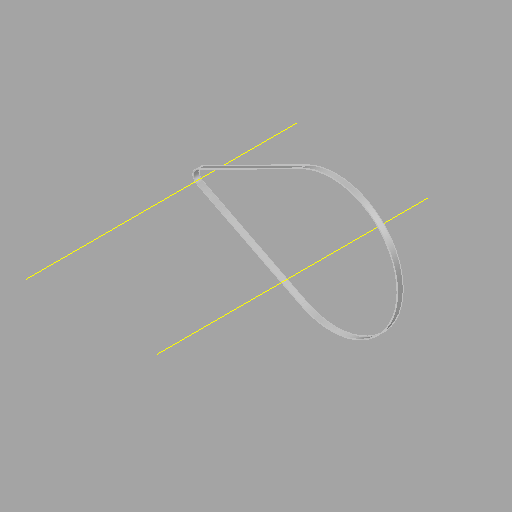
# Autodesk Inventor part: Synchronous Belt
Saved by Autodesk Inventor 2025.2 (Build 292293000, 293)
## iProperties
CustomPartVersion: 1
Created: 2025-04-10
Part Number: Synchronous Belt
Material: Rubber
Document SubType Name: Modeling
Designer: Tiago
Density: 1 g/cm^3
Appearance: Rubber - Black - Version 1.1
Author: Tiago
Autodesk Inventor part; units mm, degrees
ref_plane "YZ Plane" through (0, 0, 0) normal (1, 0, 0) x (0, 1, 0)
ref_plane "XZ Plane" through (0, 0, 0) normal (0, 1, 0) x (-1, 0, 0)
ref_plane "XY Plane" through (0, 0, 0) normal (0, 0, 1) x (1, 0, 0)
sketch "Sketch Path" plane through (0, 0, 0) normal (0, 0, 1) x (1, 0, 0)
  arc A0 (-3.5983, 7.0977) -> (-3.5983, -7.0977) centre (0, 0) ccw
  arc A1 (108.4052, -63.8797) -> (108.4052, 63.8797) centre (140.79, 0) ccw
  line L0 (108.4052, -63.8797) -> (-3.5983, -7.0977)
  line L1 (-3.5983, 7.0977) -> (108.4052, 63.8797)
  constraints: 4 end point, 4 point on circle, 2 centre point
ref_plane "Cross Section Plane" through (-3.5983, -7.0977, 0) normal (0.8919283, -0.4521768, 0) x (0, 0, 1)
ref_plane "Work Plane2" through (0, 0, 0) normal (-1, 0, 0) x (0, 0, 1)
ref_plane "Work Plane3" through (140.79, 0, 0) normal (-0.8960525, -0.443948, 0) x (0, 0, 1)
sketch "Cross Section" plane through (-3.5983, -7.0977, 0) normal (0.8919283, -0.4521768, 0) x (0, 0, 1)
  line L0 (-3, 0.3) -> (3, 0.3)
  line L1 (3, 0.3) -> (3, -0.3)
  line L2 (3, -0.3) -> (-3, -0.3)
  line L3 (-3, -0.3) -> (-3, 0.3)
  line L4 (-3, 0) -> (3, 0) construction
  point P0 (0, 0)
  point P1 (0, 0)
  dimension "d0" = 6
  dimension "d4" = 0.3
  dimension "d5" = 0.3
  constraints: 10 end point, 3 midpoint, 2 parallel, 1 coincident, 1 horizontal, 1 perpendicular, 1 other
  measures "d0" distance between parallel lines of L1 L3
  measures "d4" distance between parallel lines of L2 L4
  measures "d5" distance between parallel lines of L4 L0
sweep "Belt" add profiles "Cross Section" path "Sketch Path" path curves L1 A1 L0 A0
equation "\"d0\" = da_B"
equation "\"d4\" = da_a"
equation "\"d5\" = da_a2"
equation "\"da_B\" = 6"
equation "\"da_pb\" = 2.5"
equation "\"da_L\" = 560.89014"
equation "\"da_a\" = 0.3"
equation "\"da_S\" = 1.5"
equation "\"da_Beta\" = 20deg"
equation "\"da_Ht\" = 0.7"
equation "\"da_H\" = 1.3"
equation "\"da_a2\" = 0.3"
body "Solid1"
